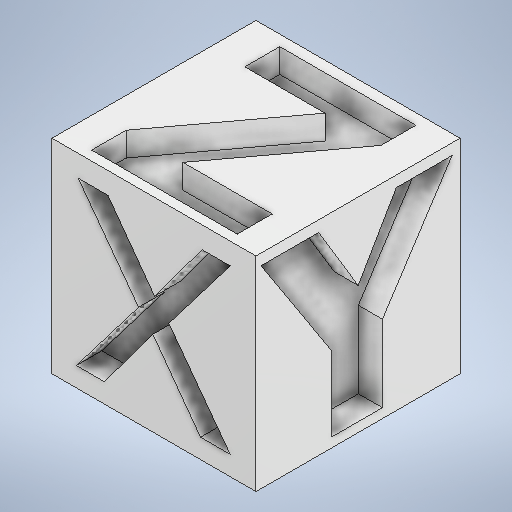
# Autodesk Inventor part: Cubo
Saved by Autodesk Inventor 2025.2 (Build 292293000, 293)
## iProperties
Created: 2025-01-18
Part Number: Cubo
Material: ABS Plastic
Document SubType Name: Modeling
Designer: Tony Dias
Density: 1.06 g/cm^3
Appearance: Smooth - White
Author: Tony Dias
## iProperties of the stored document Cubo_3DPrint.ipt
Created: 2025-01-18
Part Number: Cubo_3DPrint
Material: Generic
Document SubType Name: Modeling
Designer: Tony Dias
Density: 1 g/cm^3
Appearance: Default
Author: Tony Dias
Autodesk Inventor part; units mm, degrees
ref_plane "YZ Plane" through (0, 0, 0) normal (1, 0, 0) x (0, 1, 0)
ref_plane "XZ Plane" through (0, 0, 0) normal (0, 1, 0) x (-1, 0, 0)
ref_plane "XY Plane" through (0, 0, 0) normal (0, 0, 1) x (1, 0, 0)
sketch "Sketch3" plane through (0, 0, 0) normal (0, 0, 1) x (1, 0, 0)
  line L0 (12.7, -12.7) -> (-12.7, -12.7)
  line L1 (-12.7, -12.7) -> (-12.7, 12.7)
  line L2 (-12.7, 12.7) -> (12.7, 12.7)
  line L3 (12.7, 12.7) -> (12.7, -12.7)
  line L4 (12.7, -12.7) -> (-12.7, 12.7) construction
  line L5 (-12.7, -12.7) -> (12.7, 12.7) construction
  point P0 (0, 0)
  dimension "d0" = 25.4
  dimension "d1" = 25.4
  constraints: 12 end point, 2 midpoint, 2 parallel, 1 horizontal, 1 perpendicular
  measures "d0" distance of L1.end L2.end
  measures "d1" distance of L0.end L1.end
extrude "Cubo" add sketch "Sketch3" along normal blind 25.4
sketch "Sketch5" plane through (0, 0, 25.4) normal (0, 0, 1) x (1, 0, 0)
  line L0 (-12.1868, 12.0555) -> (12.0292, 12.0555) construction
  line L1 (12.0292, 12.0555) -> (12.0292, -12.3181) construction
  line L2 (12.0292, -12.3181) -> (-12.1868, -12.3181) construction
  line L3 (-12.1868, -12.3181) -> (-12.1868, 12.0555) construction
  line L4 (9.4966, -10.2913) -> (5.7916, -10.2913)
  line L5 (5.7916, -10.2913) -> (-0.1365, -2.1567)
  line L6 (-0.1365, -2.1567) -> (-6.1633, -10.2913)
  line L7 (-6.1633, -10.2913) -> (-9.6707, -10.2913)
  line L8 (-9.6707, -10.2913) -> (-1.9149, -0.1313)
  line L9 (-1.9149, -0.1313) -> (-9.4402, 10.0287)
  line L10 (-9.4402, 10.0287) -> (-5.7352, 10.0287)
  line L11 (-5.7352, 10.0287) -> (0.0776, 2.0588)
  line L12 (0.0776, 2.0588) -> (5.9892, 10.0287)
  line L13 (5.9892, 10.0287) -> (9.4966, 10.0287)
  line L14 (9.4966, 10.0287) -> (1.856, 0.0169)
  line L15 (1.856, 0.0169) -> (9.4966, -10.2913)
  point P0 (0, 0)
  constraints: 2 other
extrude "X" cut sketch "Sketch5" against normal blind 3.175
sketch "Esboço9" plane through (12.7, -12.7, 0) normal (1, 0, 0) x (0, 0, -1)
  line L0 (-24.9757, 24.9816) -> (-0.1587, 24.9816) construction
  line L1 (-0.1587, 24.9816) -> (-0.1587, 0.228) construction
  line L2 (-0.1587, 0.228) -> (-24.9757, 0.228) construction
  line L3 (-24.9757, 0.228) -> (-24.9757, 24.9816) construction
  line L4 (-0.989, 24.0348) -> (-9.6587, 10.7152)
  line L5 (-9.6587, 10.7152) -> (-9.6587, 1.1748)
  line L6 (-9.6587, 1.1748) -> (-15.9573, 1.1748)
  line L7 (-15.9573, 1.1748) -> (-15.9573, 10.4374)
  line L8 (-15.9573, 10.4374) -> (-24.7752, 24.0348)
  line L9 (-24.7752, 24.0348) -> (-17.606, 24.0348)
  line L10 (-17.606, 24.0348) -> (-12.6783, 15.8652)
  line L11 (-12.6783, 15.8652) -> (-7.9359, 24.0348)
  line L12 (-7.9359, 24.0348) -> (-0.989, 24.0348)
  point P0 (0, 12.7)
  constraints: 2 other
extrude "Extrusão6" cut sketch "Esboço9" against normal blind 3
sketch "Esboço10" plane through (-12.7, 12.7, 0) normal (0, 1, 0) x (1, 0, 0)
  line L0 (0.3012, -0.2854) -> (25.0988, -0.2854) construction
  line L1 (25.0988, -0.2854) -> (25.0988, -25.2732) construction
  line L2 (25.0988, -25.2732) -> (0.3012, -25.2732) construction
  line L3 (0.3012, -25.2732) -> (0.3012, -0.2854) construction
  line L4 (21.8699, -24.2093) -> (3.7524, -24.2093)
  line L5 (3.7524, -24.2093) -> (3.7524, -19.93)
  line L6 (3.7524, -19.93) -> (14.2932, -5.7027)
  line L7 (14.2932, -5.7027) -> (4.3081, -5.7027)
  line L8 (4.3081, -5.7027) -> (4.3081, -1.3493)
  line L9 (4.3081, -1.3493) -> (21.2586, -1.3493)
  line L10 (21.2586, -1.3493) -> (21.2586, -5.7027)
  line L11 (21.2586, -5.7027) -> (10.7549, -19.8559)
  line L12 (10.7549, -19.8559) -> (21.8699, -19.8559)
  line L13 (21.8699, -19.8559) -> (21.8699, -24.2093)
  point P0 (12.7, 0)
  constraints: 2 other
extrude "Extrusão7" cut sketch "Esboço10" against normal blind 3
body "Solid1"
